Autodesk Fusion 360 part; units mm, degrees
(part 2 of 2)
  measures "d50" radius of A316
  measures "d51" radius of A317
  measures "d53" radius of A318
  measures "d54" radius of A319
  measures "d55" radius of A320
  measures "d56" radius of A321
  measures "d57" radius of A322
  measures "d87" radius of A323
  measures "d88" radius of A324
  measures "d90" radius of A325
  measures "d91" radius of A326
  measures "d92" radius of A327
  measures "d100" radius of A328
  measures "d101" radius of A329
  measures "d102" radius of A330
  measures "d103" radius of A331
  measures "d104" radius of A332
  measures "d105" radius of A333
  measures "d113" radius of A334
  measures "d114" radius of A335
  measures "d115" radius of A336
  measures "d116" radius of A337
  measures "d117" radius of A338
  measures "d118" radius of A339
extrude "Extrude1" add sketch "kbplate" along normal blind 1.5 contours L299 L301 L303 L304 L305 L306 L307 L308 A300 A301 A302 A303 A304 A305 L325 A325 A326 L326 L327 L328 L329 L330 L331 L332 A328 A329 A330 A331 A332 A333 | L299 L300 L301 L308 A298 A299 A300 L318 L319 L320 A316 A317 A318 L325 A325 A327 | L299 L300 L301 A298 A299 L326 L327 L328 L329 L330 L331 L332 A328 A329 A330 A331 A332 A333 makes body 1 in component "Top_Left"
extrude "Extrude2" add sketch "kbplate" along normal blind 7.5 from surface at 1.5 contours L299 L300 L301 L308 A298 A299 A300 L318 L319 L320 A316 A317 A318 L325 A325 A327 bodies 1 in component "Top_Left"
extrude "Extrude1'" add sketch "kbplate" along normal blind 1.5 separate body contours L302 L309 L311 A313 A315 L333 L334 L335 L336 L337 L338 L339 A334 A335 A336 A337 A338 A339 | L302 L309 L310 L311 L317 A312 A313 A314 A315 L321 L322 L323 A319 A320 A321 A322 | L309 L310 L311 L312 L313 L314 L315 L316 L317 A306 A307 A308 A309 A310 A311 A312 A314 L333 L334 L335 L336 L337 L338 L339 A334 A335 A336 A337 A338 A339 makes body 2 in component "Top_Right"
extrude "Extrude2'" add sketch "kbplate" along normal blind 7.5 from surface at 1.5 contours L302 L309 L310 L311 L317 A312 A313 A314 A315 L321 L322 L323 A319 A320 A321 A322 bodies 2 in component "Top_Right"
extrude "Extrude1''" add sketch "kbplate" against normal blind 9.6 separate body contours L299 L301 L303 L304 L305 L306 L307 L308 A300 A301 A302 A303 A304 A305 L325 A325 A326 L326 L327 L328 L329 L330 L331 L332 A328 A329 A330 A331 A332 A333 | L299 L300 L301 L308 A298 A299 A300 L318 L319 L320 A316 A317 A318 L325 A325 A327 makes body 3 in component "Bottom_Left"
extrude "Extrude2''" add sketch "kbplate" against normal blind 1 from surface at -9.6 contours A6 A11 L11 A31 L29 A37 L40 L43 | L8 A13 A17 A30 L31 L32 L34 A46 | L9 A20 A27 L30 A36 L39 A47 L45 | A14 L14 L21 L22 A33 L36 A42 A48 | A16 A18 L23 L33 L35 A39 L41 A43 | L15 A29 L27 L38 A41 A45 L44 A49 | L25 L26 A35 A38 L37 A40 L42 A44 | L52 A53 L56 L58 A69 A79 L71 A83 | A55 L55 A70 A78 A85 L89 L93 L105 | L67 L80 L88 A93 A95 A100 L95 A104 | A74 L84 L86 A94 L99 A109 L102 A110 | L83 A96 L96 A103 L97 A105 L98 A114 | L87 L91 A101 A102 A106 A107 L101 L103 | A98 L94 A118 A122 L120 L123 A135 L125 | A99 L115 A126 L124 L130 L133 A137 A142 | A121 A134 L128 A138 L142 A145 L148 L176 | A146 L147 L150 L156 A154 A155 L164 A166 | L149 L152 L161 A158 A163 L174 A174 A176 | L151 A151 A157 A160 A167 L170 L172 L175 | L153 A156 A159 L163 A164 L169 A170 L173 | L157 A153 L162 L165 L167 A165 A172 A175 | L159 L160 A184 A187 A188 L199 L204 A207 | A178 A182 A189 L193 L194 L196 A198 L202 | A200 A202 A204 L207 L209 L210 A233 L235 | A209 A212 L211 L220 A222 L222 A236 L237 | L205 A217 A224 A225 A229 L228 L231 L234 | L208 L216 A220 L229 L233 A232 A235 A238 | A215 L217 L218 A221 A227 A228 L230 L236 | A242 L242 A247 L256 A260 A268 L268 L298 | L240 A249 L253 A257 L267 A275 L283 A286 | A243 L250 A254 L264 A267 A270 L278 L296 | L241 A246 A252 L252 A274 L290 L292 A293 | L243 A253 L251 A261 A269 L273 A287 L291 | L245 A263 A271 L269 L295 L324 A323 A324 | A248 L249 L255 A264 L277 L282 A284 A292 | L299 L301 L303 L304 L305 L306 L307 L308 A300 A301 A302 A303 A304 A305 L325 A325 A326 L326 L327 L328 L329 L330 L331 L332 A328 A329 A330 A331 A332 A333 | L299 L300 L301 L308 A298 A299 A300 L318 L319 L320 A316 A317 A318 L325 A325 A327 | L299 L300 L301 A298 A299 L326 L327 L328 L329 L330 L331 L332 A328 A329 A330 A331 A332 A333 bodies 3 in component "Bottom_Left"
extrude "Extrude1'''" add sketch "kbplate" against normal blind 9.6 separate body contours L302 L309 L310 L311 L317 A312 A313 A314 A315 L321 L322 L323 A319 A320 A321 A322 | L309 L310 L311 L312 L313 L314 L315 L316 L317 A306 A307 A308 A309 A310 A311 A312 A314 L333 L334 L335 L336 L337 L338 L339 A334 A335 A336 A337 A338 A339 makes body 4 in component "Bottom_Right"
extrude "Extrude2'''" add sketch "kbplate" against normal blind 1 from surface at -9.6 contours L0 L1 A26 A276 L281 A288 A291 L294 | A0 L2 L6 L10 A21 L28 A283 A289 | A1 L4 A8 A19 L19 A25 L270 L285 | A2 A9 A12 A15 L24 L48 L68 L70 | L3 L238 A259 A277 L279 A285 A294 L297 | A3 A5 L12 L20 A28 A278 L284 L287 | A4 L5 A10 L13 L18 A23 A24 L280 | A7 L7 L271 L276 L289 A290 A295 A296 | A22 A32 L272 A279 A281 L275 L286 L293 | L16 L17 A34 L274 A280 A282 L288 A297 | L46 L50 L51 A52 A56 L59 A62 A81 | L47 L49 A54 L53 A58 A65 A68 L72 | A50 A57 L62 L63 A63 L65 A64 L78 | A51 L57 L61 L66 A72 A75 A76 L79 | L54 A60 L60 A66 A77 L73 L74 A84 | A59 A61 L64 A82 L75 L76 L77 A86 | A67 A71 L69 L81 A90 A92 L104 L109 | A73 A87 A89 L85 L92 A111 L106 L108 | A80 L90 A97 L100 A113 L107 A115 L110 | A88 L82 A91 A108 A112 L119 L122 L144 | L111 A127 A128 A139 A140 L140 L141 L143 | L112 A116 A119 L118 A124 A131 L126 L127 | L113 A117 L114 A125 A129 L121 L131 A143 | A120 L116 A130 A132 L134 L136 L137 A144 | L117 A123 A133 A136 L135 L138 L139 A141 | L129 L146 A147 A149 L155 L166 A168 A171 | L132 L145 A150 L154 A152 A161 L168 A169 | A148 A162 L171 A173 A177 L182 L186 L201 | L158 L177 L188 A191 L195 A196 A201 A203 | L178 L184 L185 A190 A192 A193 L198 A195 | L179 A181 A183 L190 L191 L197 A199 A206 | A179 A180 L183 L187 L189 A185 L192 A194 | L180 L181 A186 A197 L200 A205 L203 A208 | L206 A211 A219 L219 L224 L232 A239 A240 | A210 A214 L215 A218 A223 L246 L257 L265 | A213 L214 L221 L223 L226 A230 A237 A241 | L212 L213 A216 A226 L225 L227 A231 A234 | L239 L247 A251 L254 A256 L260 A266 A272 | A244 A250 L258 L261 L263 A265 L266 A273 | A245 L244 L248 A255 L259 A258 A262 L262 | L302 L309 L311 A313 A315 L333 L334 L335 L336 L337 L338 L339 A334 A335 A336 A337 A338 A339 | L302 L309 L310 L311 L317 A312 A313 A314 A315 L321 L322 L323 A319 A320 A321 A322 | L309 L310 L311 L312 L313 L314 L315 L316 L317 A306 A307 A308 A309 A310 A311 A312 A314 L333 L334 L335 L336 L337 L338 L339 A334 A335 A336 A337 A338 A339 bodies 4 in component "Bottom_Right"
component "Top_Left" placed x (1, 0, 0) y (0, 1, 0) z (0, 0, 1) at (0, 0, 0)
component "Top_Right" placed x (1, 0, 0) y (0, 1, 0) z (0, 0, 1) at (0, 0, 0)
component "Bottom_Left" placed x (1, 0, 0) y (0, 1, 0) z (0, 0, 1) at (0, 0, 0)
component "Bottom_Right" placed x (1, 0, 0) y (0, 1, 0) z (0, 0, 1) at (0, 0, 0)
